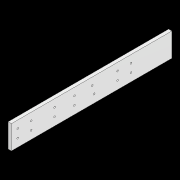
# Autodesk Inventor part: BackWallUHMW
Saved by Autodesk Inventor 2021 (Build 250183000, 183)
## iProperties
Created: 2021-03-10
Part Number: BackWallUHMW
Material: UHMW, White
Document SubType Name: Modeling
Designer: Dylan
Density: 0.94 g/cm^3
Appearance: Smooth - White
Mass: 2246.51 g
Surface Area: 2998.81 cm^2
Volume: 2389.9 cm^3
Author: Dylan
Autodesk Inventor part; units mm, degrees
ref_plane "YZ Plane" through (0, 0, 0) normal (1, 0, 0) x (0, 1, 0)
ref_plane "XZ Plane" through (0, 0, 0) normal (0, 1, 0) x (-1, 0, 0)
ref_plane "XY Plane" through (0, 0, 0) normal (0, 0, 1) x (1, 0, 0)
sketch "Sketch1" plane through (0, 0, 0) normal (1, 0, 0) x (0, 1, 0)
  line L0 (-3.175, 0) -> (133.35, 0)
  line L1 (133.35, 0) -> (133.35, -927.1)
  line L2 (133.35, -927.1) -> (-3.175, -927.1)
  line L3 (-3.175, -927.1) -> (-3.175, 0)
  point P0 (133.35, 0)
  dimension "d1" = 927.1
  constraints: 8 end point, 2 parallel, 1 horizontal, 1 perpendicular, 3 other
  measures "d1" distance of L1.end L0.end
extrude "Extrusion1" add sketch "Sketch1" along normal blind 19.05
sketch "Sketch2" plane through (0, 0, 0) normal (-1, 0, 0) x (0, 0, 1)
  circle A0 centre (-114.3, 90.4875) radius 5.0419 projected
  circle A1 centre (-114.3, 42.8625) radius 5.0419 projected
  circle A2 centre (-36.5125, 90.4875) radius 5.0419 projected
  circle A3 centre (-36.5125, 42.8625) radius 5.0419 projected
  circle A4 centre (-249.555, 90.4875) radius 5.0419 projected
  circle A5 centre (-249.555, 42.8625) radius 5.0419 projected
  circle A6 centre (-363.855, 90.4875) radius 5.0419 projected
  circle A7 centre (-363.855, 42.8625) radius 5.0419 projected
  circle A8 centre (-467.0425, 90.4875) radius 5.0419 projected
  circle A9 centre (-478.155, 42.8625) radius 5.0419 projected
  circle A10 centre (-613.41, 90.4875) radius 5.0419 projected
  circle A11 centre (-613.41, 42.8625) radius 5.0419 projected
  circle A12 centre (-691.1975, 90.4875) radius 5.0419 projected
  circle A13 centre (-691.1975, 42.8625) radius 5.0419 projected
  point P0 (0, 0)
hole "Hole1" at (0, 90.4875, -691.1975) at (0, 42.8625, -691.1975) at (0, 90.4875, -613.41) at (0, 42.8625, -613.41) at (0, 90.4875, -467.0425) at (0, 42.8625, -478.155) at (0, 90.4875, -363.855) at (0, 42.8625, -363.855) at (0, 90.4875, -249.555) at (0, 42.8625, -249.555) at (0, 90.4875, -114.3) at (0, 42.8625, -114.3) at (0, 90.4875, -36.5125) at (0, 42.8625, -36.5125) direction (1, 0, 0) diameter 10.0838 end through all clearance for "Hex Head Bolt" size "3/8" standard "Ansi Unified Screw Threads"
body "Solid1"
